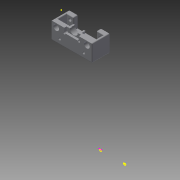
# Autodesk Inventor part: connector for board
Saved by Autodesk Inventor 2014 (Build 180170000, 170)
## iProperties
Created: 2014-01-08
Part Number: connector for board
Material: Generic
Document SubType Name: Modeling
Designer: bvjohn
Density: 1 g/cm^3
Appearance: Default
Author: bvjohn
Autodesk Inventor part; units mm, degrees
ref_plane "Work Plane1" through (0, 0, 0) normal (0, 0, 1) x (1, 0, 0)
sketch "Sketch1" plane through (0, 0, 0) normal (0, 0, 1) x (1, 0, 0)
  circle A0 centre (82.55, -115.8875) radius 1.98374
  circle A1 centre (44.45, -115.8875) radius 1.98374
  arc A2 (48.498358, -127.623507) -> (46.998508, -126.123358) centre (48.498508, -126.123507) ccw
  arc A3 (79.998507, -126.126642) -> (78.498358, -127.626492) centre (78.498507, -126.126492) ccw
  arc A4 (78.501642, -94.626493) -> (80.001492, -96.126642) centre (78.501492, -96.126493) ccw
  arc A5 (47.001493, -96.123358) -> (48.501642, -94.623508) centre (48.501493, -96.123508) ccw
  line L0 (84.502089, -90.12709) -> (42.50209, -90.122911)
  line L1 (42.50209, -90.122911) -> (42.497911, -132.12291)
  line L2 (84.49791, -132.127089) -> (84.502089, -90.12709)
  line L3 (42.497911, -132.12291) -> (84.49791, -132.127089)
  circle A6 centre (63.5, -111.125) radius 14.28115
  circle A7 centre (63.5, -111.125) radius 14.28115
  circle A8 centre (82.55, -115.8875) radius 1.98374
  circle A9 centre (44.45, -115.8875) radius 1.98374
  line L4 (38.347802, -111.125) -> (49.21885, -111.125)
  line L5 (49.21885, -111.125) -> (49.21885, -132.123579)
  line L6 (49.21885, -132.123579) -> (38.347802, -132.123579)
  line L7 (38.347802, -132.123579) -> (38.347802, -111.125)
  line L8 (88.909206, -111.125) -> (77.78115, -111.125)
  line L9 (77.78115, -111.125) -> (77.78115, -132.126421)
  line L10 (77.78115, -132.126421) -> (88.909206, -132.126421)
  line L11 (88.909206, -132.126421) -> (88.909206, -111.125)
  line L12 (49.21885, -132.123579) -> (77.78115, -132.123579)
  line L13 (77.78115, -132.123579) -> (77.78115, -125.40615)
  line L14 (77.78115, -125.40615) -> (49.21885, -125.40615)
  line L15 (49.21885, -125.40615) -> (49.21885, -132.123579)
  point P0 (0, 0)
  constraints: 24 end point, 6 parallel, 5 horizontal, 3 centre point, 3 coincident, 3 concentric, 3 perpendicular, 3 point on line, 3 tangent, 2 vertical
extrude "Extrusion1" add sketch "Sketch1" along normal blind 5 contours A0 L2 L8 L11 L10 | A0 L2 L3 L9 L8 | L5 L3 L1 A1 L4 | L14 A3 L9 L12 L5 A2 | L1 A1 L6 L7 L4 | L14 L9 A3 | A2 L5 L14 picked at (77.689311, -126.700283) picked at (49.3103, -126.697213)
sketch "Sketch2" plane through (0, 0, 5) normal (0, 0, 1) x (1, 0, 0)
  circle A0 centre (44.45, -115.8875) radius 1.98374
  circle A1 centre (82.55, -115.8875) radius 1.98374
  line L0 (88.909206, -132.126421) -> (88.909206, -111.125)
  line L1 (88.909206, -111.125) -> (77.78115, -111.125)
  line L2 (49.21885, -111.125) -> (38.347802, -111.125)
  line L3 (38.347802, -132.123579) -> (88.909206, -132.123579)
  line L4 (88.909206, -132.123579) -> (88.909206, -125.40615)
  line L5 (88.909206, -125.40615) -> (38.347802, -125.40615)
  line L6 (38.347802, -125.40615) -> (38.347802, -132.123579)
  line L7 (88.909206, -125.40615) -> (86.369206, -125.40615)
  line L8 (86.369206, -125.40615) -> (86.369206, -111.125)
  line L9 (86.369206, -111.125) -> (88.909206, -111.125)
  line L10 (88.909206, -111.125) -> (88.909206, -125.40615)
  line L11 (38.347802, -125.40615) -> (40.887802, -125.40615)
  line L12 (40.887802, -125.40615) -> (40.887802, -111.125)
  line L13 (40.887802, -111.125) -> (38.347802, -111.125)
  line L14 (38.347802, -111.125) -> (38.347802, -125.40615)
  circle A2 centre (44.45, -115.8875) radius 4.7625
  circle A3 centre (82.55, -115.8875) radius 4.7625
  point P0 (0, 0)
  dimension "d4" = 2.54
  dimension "d5" = 2.54
  constraints: 24 end point, 6 parallel, 4 horizontal, 3 perpendicular, 3 point on line, 2 centre point, 2 coincident, 2 tangent
  measures "d4" distance of L8.end L9.end
  measures "d5" distance of L13.end L12.end
extrude "Extrusion2" add sketch "Sketch2" along normal blind 11.5 contours L3 L6 L5 L0 | L5 L8 A3 L1 L0 | L14 L2 L12 A2 L5 | L8 A3 | A2 L12 picked at (86.541199, -116.544731) picked at (40.669942, -116.626014)
sketch "Sketch3" plane through (0, 0, 16.5) normal (0, 0, 1) x (1, 0, 0)
  line L0 (38.347802, -132.123579) -> (88.909206, -132.123579)
  line L1 (88.909206, -132.123579) -> (88.909206, -111.125)
  line L2 (88.909206, -111.125) -> (86.369206, -111.125)
  line L3 (86.369206, -111.125) -> (86.369206, -125.40615)
  line L4 (86.369206, -125.40615) -> (40.887802, -125.40615)
  line L5 (40.887802, -125.40615) -> (40.887802, -111.125)
  line L6 (40.887802, -111.125) -> (38.347802, -111.125)
  line L7 (38.347802, -111.125) -> (38.347802, -132.123579)
  arc A0 (48.498358, -127.623507) -> (46.998508, -126.123358) centre (48.498508, -126.123507) ccw
  line L8 (48.501493, -96.123508) -> (47.001493, -96.123358)
  line L9 (48.501642, -94.623508) -> (48.501493, -96.123508)
  arc A1 (47.001493, -96.123358) -> (48.501642, -94.623508) centre (48.501493, -96.123508) ccw
  line L10 (78.498358, -127.626492) -> (78.498507, -126.126492)
  arc A2 (79.998507, -126.126642) -> (78.498358, -127.626492) centre (78.498507, -126.126492) ccw
  line L11 (78.498507, -126.126492) -> (79.998507, -126.126642)
  line L12 (80.001492, -96.126642) -> (78.501492, -96.126493)
  arc A3 (78.501642, -94.626493) -> (80.001492, -96.126642) centre (78.501492, -96.126493) ccw
  line L13 (78.501492, -96.126493) -> (78.501642, -94.626493)
  line L14 (46.998508, -126.123358) -> (48.498508, -126.123507)
  arc A4 (48.498358, -127.623507) -> (46.998508, -126.123358) centre (48.498508, -126.123507) ccw
  line L15 (48.498508, -126.123507) -> (48.498358, -127.623507)
  line L16 (42.50209, -90.122911) -> (42.497911, -132.12291)
  line L17 (42.497911, -132.12291) -> (84.49791, -132.127089)
  line L18 (84.49791, -132.127089) -> (84.502089, -90.12709)
  line L19 (84.502089, -90.12709) -> (42.50209, -90.122911)
  line L20 (38.347802, -132.123579) -> (88.909206, -132.123579)
  circle A5 centre (48.498508, -126.123507) radius 1.5
  circle A6 centre (78.498507, -126.126492) radius 1.5
  line L21 (84.49791, -132.127089) -> (84.499453, -116.62709)
  line L22 (84.499453, -116.62709) -> (72.499453, -116.625895)
  line L23 (42.497911, -132.12291) -> (42.499453, -116.62291)
  line L24 (42.499453, -116.62291) -> (54.499453, -116.624104)
  circle A7 centre (54.499453, -116.624104) radius 1.5
  circle A8 centre (72.499453, -116.625895) radius 1.5
  line L25 (38.347802, -111.125) -> (88.909206, -111.125)
  line L26 (88.909206, -111.125) -> (88.909206, -132.123579)
  line L27 (88.909206, -132.123579) -> (38.347802, -132.123579)
  line L28 (38.347802, -132.123579) -> (38.347802, -111.125)
  line L29 (38.347802, -111.125) -> (88.909206, -111.125)
  line L30 (88.909206, -111.125) -> (88.909206, -132.123579)
  line L31 (88.909206, -132.123579) -> (38.347802, -132.123579)
  line L32 (38.347802, -132.123579) -> (38.347802, -111.125)
  point P0 (0, 0)
  dimension "d10" = 15.5
  dimension "d11" = 12
  dimension "d12" = 15.5
  dimension "d13" = 12
  dimension "d14" = 3
  dimension "d15" = 3
  constraints: 26 end point, 4 coincident, 4 parallel, 4 perpendicular, 3 horizontal, 2 centre point, 2 point on line, 1 vertical, 6 other
  measures "d10" distance of L17.end L21.end
  measures "d11" distance of L21.end L22.end
  measures "d12" distance of L16.end L23.end
  measures "d13" distance of L23.end L24.end
  measures "d14" diameter of A7
  measures "d15" diameter of A8
sketch "Sketch3 outline for Extrusion3" plane through (0, 0, 16.5) normal (0, 0, 1) x (1, 0, 0)
  line L0 (88.909206, -132.123579) -> (88.909206, -111.125)
  line L1 (88.909206, -111.125) -> (38.347802, -111.125)
  line L2 (38.347802, -111.125) -> (38.347802, -132.123579)
  line L3 (38.347802, -132.123579) -> (88.909206, -132.123579)
  circle A0 centre (72.499453, -116.625895) radius 1.5
  circle A1 centre (54.499453, -116.624104) radius 1.5
  arc A2 (79.814223, -125.40615) -> (77.182792, -125.40615) centre (78.498507, -126.126492) ccw
  line L4 (79.814223, -125.40615) -> (77.182792, -125.40615)
  arc A3 (49.815853, -125.40615) -> (47.181162, -125.40615) centre (48.498508, -126.123507) ccw
  line L5 (49.815853, -125.40615) -> (47.181162, -125.40615)
extrude "Extrusion3" add sketch "Sketch3 outline for Extrusion3" along normal blind 5.3
sketch "Sketch4" plane through (0, 0, 21.8) normal (0, 0, 1) x (1, 0, 0)
  line L0 (77.182792, -125.40615) -> (79.814223, -125.40615)
  arc A0 (79.814223, -125.40615) -> (77.182792, -125.40615) centre (78.498507, -126.126492) ccw
  line L1 (47.181162, -125.40615) -> (49.815853, -125.40615)
  arc A1 (49.815853, -125.40615) -> (47.181162, -125.40615) centre (48.498508, -126.123507) ccw
  circle A2 centre (78.498507, -126.126492) radius 1.5
  circle A3 centre (48.498508, -126.123507) radius 1.5
  point P0 (0, 0)
  constraints: 2 coincident, 1 centre point, 4 other
extrude "Extrusion4" cut sketch "Sketch4" against normal blind 15.3 contours L0 A2 | L1 A3
sketch "Sketch5" plane through (0, 0, 6.5) normal (0, 0, 1) x (1, 0, 0)
  line L0 (77.182792, -125.40615) -> (79.814223, -125.40615)
  arc A0 (47.181162, -125.40615) -> (49.815853, -125.40615) centre (48.498508, -126.123507) ccw
  arc A1 (77.182792, -125.40615) -> (79.814223, -125.40615) centre (78.498507, -126.126492) ccw
  point P0 (0, 0)
sketch "Sketch6" plane through (49.21885, -125.40615, 0) normal (0, 1, 0) x (1, 0, 0)
  line L0 (37.150356, -16.5) -> (30.595373, -16.5)
  line L1 (-2.037688, -16.5) -> (-8.331048, -16.5)
  line L2 (27.963942, -16.5) -> (0.597003, -16.5)
  line L3 (-2.037688, -16.5) -> (-5.037688, -16.5)
  line L4 (0.597003, -16.5) -> (3.597003, -16.5)
  line L5 (-5.037688, -16.5) -> (3.597003, -16.5)
  line L6 (3.597003, -16.5) -> (3.597003, -11.5)
  line L7 (3.597003, -11.5) -> (-5.037688, -11.5)
  line L8 (-5.037688, -11.5) -> (-5.037688, -16.5)
  line L9 (27.963942, -16.5) -> (24.963942, -16.5)
  line L10 (30.595373, -16.5) -> (33.595373, -16.5)
  line L11 (33.595373, -16.5) -> (24.963942, -16.5)
  line L12 (24.963942, -16.5) -> (24.963942, -11.5)
  line L13 (24.963942, -11.5) -> (33.595373, -11.5)
  line L14 (33.595373, -11.5) -> (33.595373, -16.5)
  point P0 (-49.21885, 0)
  point P1 (24.963942, -14)
  dimension "d20" = 3
  dimension "d21" = 3
  dimension "d22" = 5
  dimension "d23" = 3
  dimension "d24" = 3
  constraints: 24 end point, 4 parallel, 4 point on line, 3 horizontal, 2 perpendicular, 1 midpoint, 1 vertical, 1 other
  measures "d20" distance of L1.start L3.end
  measures "d21" distance of L2.end L4.end
  measures "d22" distance of L6.end L5.end
  measures "d23" distance of L2.start L9.end
  measures "d24" distance of L0.end L10.end
extrude "Extrusion5" cut sketch "Sketch6" against normal blind 152.4
sketch "Sketch7" plane through (0, 0, 16.5) normal (0, 0, -1) x (-1, 0, 0)
  circle A0 centre (-63.5, -111.125) radius 5 projected
  circle A1 centre (-63.5, -111.125) radius 5
  point P0 (0, 0)
  constraints: 1 centre point, 1 coincident, 1 concentric
extrude "Extrusion6" cut sketch "Sketch7" against normal blind 2.55
sketch "Sketch8" plane through (0, 0, 21.8) normal (0, 0, 1) x (1, 0, 0)
  circle A0 centre (54.499453, -116.624104) radius 1.5
  circle A1 centre (72.499453, -116.625895) radius 1.5
  line L0 (88.909206, -111.125) -> (38.347802, -111.125)
  line L1 (54.499453, -116.624104) -> (54.499453, -111.125)
  line L2 (72.499453, -116.625895) -> (72.499453, -111.125)
  line L3 (72.499453, -116.625895) -> (54.499453, -116.624104)
  line L4 (54.499453, -111.125) -> (72.499453, -111.125)
  point P0 (0, 0)
  constraints: 8 end point, 2 perpendicular, 2 point on line, 1 parallel
ref_plane "Work Plane2" through (57.952157, -116.672843, 19.01) normal (0, 0, 1) x (0.9932069, -0.1163617, 0)
extrude "Extrusion7" cut sketch "Sketch8" against normal up to surface (2.79 mm away) contours L3 L1 A0 | A0 L1 L0 L2 A1 L3 | A1 L2 L3 picked at (55.202114, -115.921443) picked at (71.658086, -116.097154)
sketch "Sketch9" plane through (0, 0, 16.5) normal (0, 0, -1) x (-1, 0, 0)
  arc A0 (-68.5, -111.125) -> (-58.5, -111.125) centre (-63.5, -111.125) ccw
  line L0 (-86.369206, -111.125) -> (-68.5, -111.125)
  line L1 (-58.5, -111.125) -> (-40.887802, -111.125)
  arc A1 (-69, -111.125) -> (-58, -111.125) centre (-63.5, -111.125) ccw
  arc A2 (-71, -111.125) -> (-56, -111.125) centre (-63.5, -111.125) ccw
  line L2 (-71, -111.125) -> (-69, -111.125)
  line L3 (-58, -111.125) -> (-56, -111.125)
  point P0 (0, 0)
  dimension "d32" = 5.5
  dimension "d33" = 7.5
  constraints: 4 end point, 4 point on circle, 2 centre point, 2 coincident, 2 collinear, 2 point on line, 1 horizontal
  measures "d32" radius of A1
  measures "d33" radius of A2
ref_plane "Work Plane3" through (57.952157, -116.672843, 12.01) normal (0, 0, -1) x (0.1163617, 0.9932069, 0)
extrude "Extrusion8" add sketch "Sketch9" along normal up to surface (4.49 mm away) contours A1 L1 A2 L0
fillet "Fillet2" radius 1 16 edges at (88.9092, -111.125, 10.9) (38.3478, -111.125, 10.9) (38.3478, -132.1236, 10.9) (88.9092, -132.1236, 13.4) (88.9092, -132.1264, 2.5) (88.9092, -121.6243, 21.8) (63.6285, -132.1236, 21.8) (38.3478, -121.6243, 21.8) (40.8878, -111.125, 10.75) (86.3692, -111.125, 10.75) (82.0752, -111.125, 5) (45.0533, -111.125, 5) (49.2188, -118.2656, 5) (49.2188, -111.125, 2.5) (77.7811, -111.125, 2.5) (77.7811, -118.2656, 5)
sketch "Sketch10" plane through (49.21885, -125.40615, 0) normal (0, 1, 0) x (1, 0, 0)
  line L0 (27.963942, -11.5) -> (27.963942, -6.5)
  line L1 (30.595373, -6.5) -> (30.595373, -11.5)
  line L2 (30.595373, -11.5) -> (33.595373, -11.5)
  line L3 (37.150356, -16.5) -> (33.595373, -16.5)
  line L4 (-5.037688, -16.5) -> (-8.331048, -16.5)
  line L5 (-2.037688, -11.5) -> (-2.037688, -6.5)
  line L6 (0.597003, -6.5) -> (0.597003, -11.5)
  line L7 (3.597003, -11.5) -> (3.597003, -16.5)
  line L8 (-5.037688, -16.5) -> (-5.037688, -11.5)
  line L9 (33.595373, -11.5) -> (33.595373, -16.5)
  line L10 (24.963942, -16.5) -> (24.963942, -11.5)
  line L11 (24.963942, -11.5) -> (22.963942, -11.5)
  line L12 (22.963942, -11.5) -> (22.963942, -9.5)
  line L13 (33.595373, -16.5) -> (35.595373, -16.5)
  line L14 (35.595373, -9.5) -> (35.595373, -16.5)
  line L15 (22.963942, -16.5) -> (22.963942, -9.5)
  line L16 (-5.037688, -16.5) -> (-7.037688, -16.5)
  line L17 (3.597003, -11.5) -> (5.597003, -11.5)
  line L18 (5.597003, -11.5) -> (5.597003, -9.5)
  line L19 (-7.037688, -9.5) -> (-7.037688, -16.5)
  line L20 (5.597003, -16.5) -> (5.597003, -9.5)
  line L21 (-2.037688, -9.5) -> (-2.037688, -11.5)
  line L22 (0.597003, -11.5) -> (0.597003, -9.5)
  line L23 (5.597003, -9.5) -> (0.597003, -9.5)
  line L24 (-2.037688, -9.5) -> (-7.037688, -9.5)
  line L25 (-5.037688, -11.5) -> (-2.037688, -11.5)
  line L26 (0.597003, -11.5) -> (3.597003, -11.5)
  line L27 (27.963942, -9.5) -> (27.963942, -11.5)
  line L28 (30.595373, -11.5) -> (30.595373, -9.5)
  line L29 (22.963942, -9.5) -> (27.963942, -9.5)
  line L30 (30.595373, -9.5) -> (35.595373, -9.5)
  line L31 (24.963942, -11.5) -> (27.963942, -11.5)
  line L32 (30.595373, -11.5) -> (33.595373, -11.5)
  line L33 (0.597003, -9.5) -> (0.597003, -11.5)
  line L34 (3.597003, -11.5) -> (3.597003, -16.5)
  line L35 (5.597003, -16.5) -> (5.597003, -9.5)
  line L36 (-2.037688, -9.5) -> (-2.037688, -11.5)
  line L37 (-5.037688, -11.5) -> (-5.037688, -16.5)
  line L38 (-5.037688, -16.5) -> (-7.037688, -16.5)
  line L39 (-7.037688, -16.5) -> (-7.037688, -9.5)
  line L40 (-2.037688, -9.5) -> (-7.037688, -9.5)
  line L41 (0.597003, -11.5) -> (3.597003, -11.5)
  line L42 (0.597003, -9.5) -> (5.597003, -9.5)
  line L43 (5.597003, -9.5) -> (5.597003, -11.5)
  line L44 (5.597003, -11.5) -> (5.597003, -16.5)
  line L45 (3.597003, -16.5) -> (5.597003, -16.5)
  line L46 (3.597003, -11.5) -> (3.597003, -16.5)
  line L47 (3.597003, -16.5) -> (5.597003, -16.5)
  line L48 (5.597003, -16.5) -> (5.597003, -9.5)
  line L49 (5.597003, -9.5) -> (0.597003, -9.5)
  line L50 (0.597003, -11.5) -> (0.597003, -9.5)
  line L51 (33.595373, -16.5) -> (30.595373, -16.5)
  line L52 (35.595373, -16.5) -> (33.595373, -16.5)
  line L53 (24.963942, -16.5) -> (22.963942, -16.5)
  line L54 (-2.037688, -16.5) -> (-5.037688, -16.5)
  line L55 (-7.037688, -16.5) -> (-5.037688, -16.5)
  line L56 (3.597003, -16.5) -> (5.597003, -16.5)
  line L57 (22.963942, -11.5) -> (24.963942, -11.5)
  line L58 (24.963942, -11.5) -> (24.963942, -16.5)
  line L59 (24.963942, -16.5) -> (22.963942, -16.5)
  line L60 (22.963942, -16.5) -> (22.963942, -11.5)
  point P0 (-49.21885, 0)
  dimension "d37" = 2
  dimension "d38" = 2
  dimension "d39" = 2
  dimension "d40" = 2
  dimension "d41" = 2
  constraints: 108 end point, 24 parallel, 18 perpendicular, 9 horizontal, 8 collinear, 8 point on line
  measures "d37" distance of L10.end L11.end
  measures "d38" distance of L11.end L12.end
  measures "d39" distance of L3.end L13.end
  measures "d40" distance of L8.start L16.end
  measures "d41" distance of L7.start L17.end
sketch "Sketch10 outline for Extrusion9" plane through (49.21885, -125.40615, 0) normal (0, 1, 0) x (1, 0, 0)
  line L0 (5.597003, -9.5) -> (0.597003, -9.5)
  line L1 (0.597003, -9.5) -> (0.597003, -11.5)
  line L2 (0.597003, -11.5) -> (3.597003, -11.5)
  line L3 (3.597003, -11.5) -> (3.597003, -16.5)
  line L4 (3.597003, -16.5) -> (5.597003, -16.5)
  line L5 (5.597003, -16.5) -> (5.597003, -9.5)
  line L6 (22.963942, -9.5) -> (22.963942, -16.5)
  line L7 (22.963942, -16.5) -> (24.963942, -16.5)
  line L8 (24.963942, -16.5) -> (24.963942, -11.5)
  line L9 (24.963942, -11.5) -> (27.963942, -11.5)
  line L10 (27.963942, -11.5) -> (27.963942, -9.5)
  line L11 (27.963942, -9.5) -> (22.963942, -9.5)
  line L12 (-7.037688, -9.5) -> (-7.037688, -16.5)
  line L13 (-2.037688, -9.5) -> (-7.037688, -9.5)
  line L14 (-2.037688, -11.5) -> (-2.037688, -9.5)
  line L15 (-5.037688, -11.5) -> (-2.037688, -11.5)
  line L16 (-5.037688, -16.5) -> (-5.037688, -11.5)
  line L17 (-7.037688, -16.5) -> (-5.037688, -16.5)
  line L18 (35.595373, -9.5) -> (30.595373, -9.5)
  line L19 (35.595373, -16.5) -> (35.595373, -9.5)
  line L20 (33.595373, -16.5) -> (35.595373, -16.5)
  line L21 (33.595373, -11.5) -> (33.595373, -16.5)
  line L22 (30.595373, -11.5) -> (33.595373, -11.5)
  line L23 (30.595373, -9.5) -> (30.595373, -11.5)
extrude "Extrusion9" add sketch "Sketch10 outline for Extrusion9" along normal blind 5
sketch "Sketch11" plane through (0, 0, 21.8) normal (0, 0, 1) x (1, 0, 0)
  circle A0 centre (44.45, -115.8875) radius 1.98374
  circle A1 centre (82.55, -115.8875) radius 1.98374
  circle A2 centre (44.45, -115.8875) radius 1.98374
  circle A3 centre (82.55, -115.8875) radius 1.98374
  circle A4 centre (44.45, -115.8875) radius 3.5
  circle A5 centre (82.55, -115.8875) radius 3.5
  point P0 (0, 0)
  dimension "d44" = 7
  dimension "d45" = 7
  constraints: 4 centre point, 4 coincident, 2 concentric
  measures "d44" diameter of A4
  measures "d45" diameter of A5
extrude "Extrusion10" cut sketch "Sketch11" against normal up to surface (5.3 mm away) contours A0 | A1 | A4 | A5
move or copy body "Move Body1" bodies to move or copy 1 copy no translate (-35.56, 109.22, 0)
body "Solid1"
